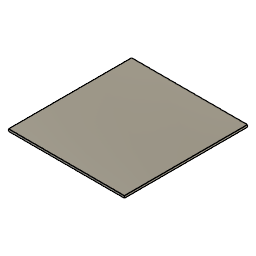
piano_inferiore_grezzo_senza_fori (Autodesk Fusion 360 design; units mm, degrees)
part number: 2026-07-13-13-55-45-167
part number: 2026-07-13-13-55-45-407
Autodesk Fusion 360 part; units mm, degrees
sketch "Schizzo1" plane through (0, 0, 0) normal (0, 0, 1) x (1, 0, 0) in component "01_Piano_inferiore_GREZZO_senza_fori"
  line L0 (-80, -85) -> (80, -85)
  line L1 (80, -85) -> (80, 85)
  line L2 (80, 85) -> (-80, 85)
  line L3 (-80, 85) -> (-80, -85)
extrude "Estrusione_Piano_inferiore" add sketch "Schizzo1" along normal blind 3 in component "01_Piano_inferiore_GREZZO_senza_fori"
component "01_Piano_inferiore_GREZZO_senza_fori" placed x (1, 0, 0) y (0, 1, 0) z (0, 0, 1) at (0, 0, 0)
equation "piano_inf_lunghezza = 170.0 mm" comment "Piano inferiore"
equation "piano_inf_larghezza = 160.0 mm" comment "Piano inferiore"
equation "piano_inf_spessore = 3.0 mm" comment "Piano inferiore"
equation "d4 = piano_inf_spessore"
named bodies: "Piano_inferiore"
